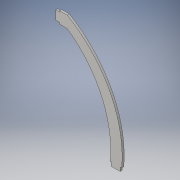
# Autodesk Inventor part: RTS gift arm
Saved by Autodesk Inventor 2016 (Build 200138000, 138)
## iProperties
Created: 2017-12-19
Part Number: RTS gift arm
Material: Generic
Document SubType Name: Modeling
Designer: student
Density: 1 g/cm^3
Appearance: Default
Author: student
Autodesk Inventor part; units mm, degrees
ref_plane "YZ Plane" through (0, 0, 0) normal (1, 0, 0) x (0, 1, 0)
ref_plane "XZ Plane" through (0, 0, 0) normal (0, 1, 0) x (-1, 0, 0)
ref_plane "XY Plane" through (0, 0, 0) normal (0, 0, 1) x (1, 0, 0)
sketch "Sketch1" plane through (0, 0, 0) normal (0, 0, 1) x (1, 0, 0)
  line L0 (-6.985, -10.16) -> (6.985, -10.16)
  line L1 (5.08, -10.16) -> (5.08, -14.732)
  line L2 (5.08, -14.732) -> (-5.588, -14.732)
  line L3 (-5.588, -14.732) -> (-5.588, -10.16)
  line L4 (-68.0064, 116.8309) -> (-68.0064, 102.8609)
  line L5 (-68.0064, 104.7659) -> (-72.5784, 104.7659)
  line L6 (-72.5784, 104.7659) -> (-72.5784, 115.4339)
  line L7 (-72.5784, 115.4339) -> (-68.0064, 115.4339)
  line L8 (-68.0064, 116.8309) -> (-58.7093, 116.8309)
  arc A0 (6.985, -10.16) -> (-58.7093, 116.8309) centre (-125.8236, 1.6238) ccw
  line L9 (-68.0064, 102.8609) -> (-58.7093, 102.8609)
  arc A1 (-6.985, -10.16) -> (-58.7093, 102.8609) centre (-129.2297, 2.2407) ccw
  point P0 (0, 0)
  point P1 (0, -10.16)
  point P2 (-68.0064, 109.8459)
  dimension "d0" = 13.97
  dimension "d2" = 10.668
  dimension "d4" = 4.572
  dimension "d5" = 13.97
  dimension "d7" = 10.668
  dimension "d8" = 4.572
  constraints: 20 end point, 4 point on circle, 4 point on line, 2 centre point, 2 horizontal, 2 midpoint, 2 parallel
  measures "d0" distance of L0.end L0.start
  measures "d2" distance of L1.end L2.end
  measures "d4" distance of L1.start L1.end
  measures "d5" distance of L4.end L4.start
  measures "d7" distance of L6.start L6.end
  measures "d8" distance of L5.start L6.start
extrude "Extrusion1" add sketch "Sketch1" along normal blind 2.54
body "Solid1"
